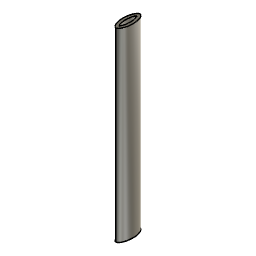
Here3 GPS Link Pole (Autodesk Fusion 360 design; units mm, degrees)
Autodesk Fusion 360 part; units mm, degrees
sketch "Sketch2" plane through (0, 0, 0) normal (0, 0, 1) x (1, 0, 0)
  spline S0 degree 3 poles (4.318, -6.6675) (4.5058, -6.6675) (4.7444, -6.6038) (5.0932, -6.2906) (5.5872, -5.8469) (6.1854, -4.8757) (6.5638, -3.5811) (7.0421, -1.9444) (7.1769, 0.1698) (6.9012, 2.0238) (6.6903, 3.4422) (6.2417, 4.6991) (5.731, 5.5084) (5.3223, 6.1561) (4.8937, 6.4913) (4.62, 6.6032) (4.3858, 6.6988) (4.2614, 6.6991) (4.0313, 6.6093) (3.7528, 6.5005) (3.3065, 6.1556) (2.884, 5.4749) (2.2706, 4.4864) (1.765, 2.8489) (1.6288, 1.0799) (1.4823, -0.8239) (1.7593, -2.8587) (2.3198, -4.3174) (2.7004, -5.3081) (3.2081, -6.0168) (3.6164, -6.354) (3.9309, -6.6137) (4.1436, -6.6675) (4.318, -6.6675) knots -3.141593 -3.141593 -3.141593 -3.141593 -2.70245 -2.70245 -2.70245 -2.080314 -2.080314 -2.080314 -1.29382 -1.29382 -1.29382 -0.692098 -0.692098 -0.692098 -0.210514 -0.210514 -0.210514 0.201462 0.201462 0.201462 0.70034 0.70034 0.70034 1.424697 1.424697 1.424697 2.204308 2.204308 2.204308 2.733774 2.733774 2.733774 3.141593 3.141593 3.141593 3.141593
  spline S1 degree 3 poles (4.3171, -4.8605) (4.4333, -4.696) (4.5656, -4.4746) (4.6935, -4.2101) (4.8394, -3.9083) (4.9801, -3.5506) (5.0965, -3.1523) (5.4971, -1.7816) (5.6294, 0.1839) (5.3892, 1.799) (5.2053, 3.0355) (4.7834, 4.1458) (4.4383, 4.6926) (4.397, 4.758) (4.3571, 4.8162) (4.3181, 4.869) knots -2.512465 -2.512465 -2.512465 -2.512465 -2.310623 -2.310623 -2.310623 -2.080314 -2.080314 -2.080314 -1.29382 -1.29382 -1.29382 -0.692098 -0.692098 -0.692098 -0.620621 -0.620621 -0.620621 -0.620621
  spline S2 degree 3 poles (4.3181, 4.869) (4.2744, 4.8099) (4.2295, 4.744) (4.1828, 4.6688) (3.8375, 4.1124) (3.421, 2.9745) (3.237, 1.7159) (3.2009, 1.4691) (3.1725, 1.2171) (3.1529, 0.9626) (3.0241, -0.7111) (3.2965, -2.5973) (3.7467, -3.7692) (3.9257, -4.2351) (4.1392, -4.6129) (4.3171, -4.8605) knots 0.620169 0.620169 0.620169 0.620169 0.70034 0.70034 0.70034 1.305947 1.305947 1.305947 1.424697 1.424697 1.424697 2.204308 2.204308 2.204308 2.515123 2.515123 2.515123 2.515123
  dimension "d18" = -1.5286
  measures "d18" distance of S0
extrude "Extrude2" add sketch "Sketch2" along normal blind 101.6
